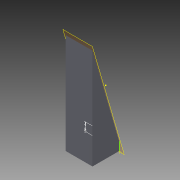
# Autodesk Inventor part: Absorber
Saved by Autodesk Inventor 2015 (Build 190159000, 159)
## iProperties
Created: 2014-07-30
Part Number: Absorber
Material: Generic
Document SubType Name: Modeling
Designer: jad211
Density: 1 g/cm^3
Appearance: Default
Author: jad211
Autodesk Inventor part; units mm, degrees
ref_plane "YZ Plane" through (0, 0, 0) normal (1, 0, 0) x (0, 1, 0)
ref_plane "XZ Plane" through (0, 0, 0) normal (0, 1, 0) x (-1, 0, 0)
ref_plane "XY Plane" through (0, 0, 0) normal (0, 0, 1) x (1, 0, 0)
sketch "Sketch1" plane through (0, 0, 0) normal (0, 1, 0) x (-1, 0, 0)
  line L0 (-8, 30) -> (8, 30)
  line L1 (8, 30) -> (8, -30)
  line L2 (8, -30) -> (-8, -30)
  line L3 (-8, -30) -> (-8, 30)
  line L4 (-8, 30) -> (8, -30) construction
  line L5 (8, 30) -> (-8, -30) construction
  point P0 (0, 0)
  dimension "d0" = 60
  dimension "d1" = 16
  constraints: 12 end point, 3 perpendicular, 2 midpoint, 1 vertical
  measures "d0" distance of L0.end L1.end
  measures "d1" distance of L1.end L2.end
extrude "Extrusion1" add sketch "Sketch1" along normal blind 16
sketch "Sketch2" plane through (0, 16, 0) normal (0, 1, 0) x (1, 0, 0)
  line L0 (8, 30) -> (-7.9475, 30)
  line L1 (-7.9475, 30) -> (-7.9475, 25)
  line L2 (-7.9475, 25) -> (8, 25)
  line L3 (8, 25) -> (8, 30)
  point P0 (0, 0)
  dimension "d4" = 5
  constraints: 8 end point
  measures "d4" distance between parallel lines of L0 L2
ref_plane "Work Plane1" through (8, 0, 30) normal (0, -0.9602, -0.2793) x (-1, 0, 0)
split "Split1" plane through (8, 0, 30) removes the side toward (0, 0.9602, 0.2793)
body "Solid1"
